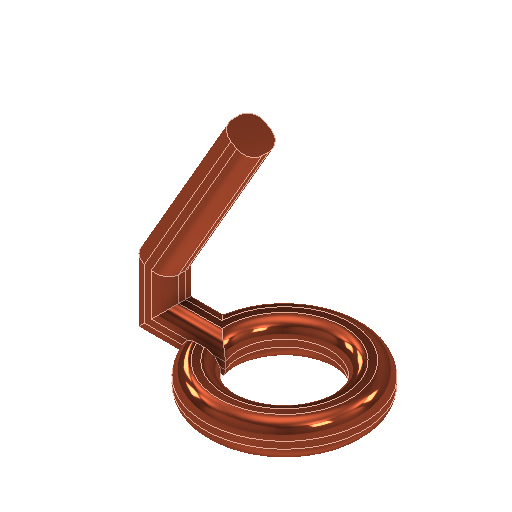
# Autodesk Inventor part: CUT_COPPER_Bottom_Cone_1,5mm_Connecting_Wire
Saved by Autodesk Inventor 2026.1 (Build 301233000, 233)
## iProperties
Created: 2025-06-19
Part Number: CUT_COPPER_Bottom_Cone_1,5mm_Connecting_Wire
Material: Generic
Document SubType Name: Modeling
Designer: User
Density: 1 g/cm^3
Appearance: Copper - Polished
Author: User
Autodesk Inventor part; units mm, degrees
ref_plane "YZ Plane" through (0, 0, 0) normal (1, 0, 0) x (0, 1, 0)
ref_plane "XZ Plane" through (0, 0, 0) normal (0, 1, 0) x (-1, 0, 0)
sketch "Sketch1" plane through (0, 0, 0) normal (0, 1, 0) x (-1, 0, 0)
  circle A0 centre (0, 0) radius 2
  circle A1 centre (0, 0) radius 3.5
  line L0 (6, 0.75) -> (3.4187, 0.75)
  line L1 (6, 0.75) -> (6, -0.75)
  line L2 (6, -0.75) -> (3.4187, -0.75)
  line L3 (3.4187, 0.75) -> (1.854, 0.75)
  line L4 (3.2692, 1.25) -> (1.5612, 1.25)
  dimension "d0" = 4
  dimension "d1" = 1.5
  dimension "d2" = 0.75
  dimension "d3" = 0.75
  dimension "d4" = 6
  dimension "d5" = 0.5
  constraints: 10 end point, 5 point on circle, 2 centre point, 2 horizontal, 1 coincident, 1 parallel, 1 perpendicular, 1 vertical
  measures "d0" diameter of A0
  measures "d1" radial gap between concentric circles of A0 A1
  measures "d2" distance from line of L0 point (0, 0)
  measures "d3" distance from line of point (0, 0) L2
  measures "d4" distance from line of point (0, 0) L1
  measures "d5" distance between parallel lines of L3 L4
extrude "Extrusion1" add sketch "Sketch1" along normal blind 1.5 contours A0 L3 A1 L4 | L0 L1 L2 A1 picked at (2.5643, 1.5047)
ref_plane "Work Plane1" through (-6, 0.6, 0.75) normal (0, 0, 1) x (1, 0, 0)
sketch "Sketch2" plane through (-6, 0.6, 0.75) normal (0, 0, 1) x (1, 0, 0)
  line L0 (0, 0.9) -> (0, 2.4)
  line L1 (0, 2.4) -> (1.5, 2.4)
  line L2 (1.5, 2.4) -> (1.5, 0.9)
  line L3 (0, 2.4) -> (3.875, 9.1117)
  line L4 (3.875, 9.1117) -> (5.174, 8.3617)
  line L5 (5.174, 8.3617) -> (1.5, 1.9981)
  line L6 (0, 0.9) -> (4.146, 0.9) projected
  point P0 (6, -0.6)
  dimension "d9" = 1.5
  dimension "d15" = 1.5
  dimension "d16" = 7
  dimension "d17" = 1.5
  dimension "d18" = 60
  constraints: 12 end point, 4 perpendicular, 1 point on line, 1 vertical
  measures "d9" distance between parallel lines of L2 L0
  measures "d15" distance between parallel lines of L5 L3
  measures "d16" distance from line of L1.end L4
  measures "d17" distance between parallel lines of L1 L6
  measures "d18" angle of L5 L6
extrude "Extrusion2" add sketch "Sketch2" against normal blind 1.5
fillet "Fillet2" radius 0.6 16 edges at (3.4903, 1.5, -0.2609) (1.7259, 1.5, -1.0107) (1.7259, 0, -1.0107) (3.4903, 0, -0.2609) (-3.927, 0, 0.75) (-4.7093, 0, -0.75) (-3.177, 1.5, 0.75) (-6, 1.5, 0.75) (-6, 1.5, -0.75) (-4.0625, 6.3558, 0.75) (-4.0625, 6.3558, -0.75) (-4.5, 2.049, 0.75) (-4.5, 2.049, -0.75) (-2.663, 5.7799, 0.75) (-2.663, 5.7799, -0.75) (-3.9593, 1.5, -0.75)
equation "\"d3\" = d2"
body "Solid1"
